Autodesk Fusion 360 part; units mm, degrees
note: some values were not read from the file. Chosen so that the rebuilt part matches the saved one: which bodies a step acts on.
(part 2 of 2)
  arc A177 (168.3933, -28.1734) -> (169.3933, -29.1734) centre (169.3933, -28.1734) ccw
  arc A178 (168.3933, -28.1734) -> (169.3933, -29.1734) centre (169.3933, -28.1734) ccw
  line L233 (31.4836, -7.7355) -> (36.2443, -10.861)
  line L234 (10.9623, -64.1171) -> (5.4942, -62.1268)
  line L235 (96.3933, -30.1734) -> (89.3933, -30.1734)
  line L236 (5.4942, -62.1268) -> (22.5952, -15.1422)
  line L237 (410.3933, -50.1734) -> (410.3933, -48.1734)
  arc A179 (386.6208, -12.1734) -> (390.6208, -16.1734) centre (386.6208, -16.1734) cw
  arc A180 (88.3933, -33.1734) -> (89.3933, -34.1734) centre (89.3933, -33.1734) ccw
  arc A181 (386.6208, -12.1734) -> (390.6208, -16.1734) centre (386.6208, -16.1734) cw
  line L238 (401.3933, -58.1734) -> (401.3933, -60.1734)
  arc A182 (96.3933, -34.1734) -> (97.3933, -33.1734) centre (96.3933, -33.1734) ccw
  arc A183 (88.3933, -23.1734) -> (89.3933, -24.1734) centre (89.3933, -23.1734) ccw
  line L239 (28.0509, -66.2863) -> (7.5421, -73.514)
  arc A184 (402.3933, -47.1734) -> (401.3933, -48.1734) centre (402.3933, -48.1734) ccw
  arc A185 (176.3933, -29.1734) -> (177.3933, -28.1734) centre (176.3933, -28.1734) ccw
  line L240 (177.3933, -22.1734) -> (177.3933, -16.1734)
  line L241 (168.3933, -22.1734) -> (168.3933, -16.1734)
  arc A186 (108.1658, -53.1734) -> (112.1658, -49.1734) centre (112.1658, -53.1734) cw
  line L242 (169.3933, -29.1734) -> (176.3933, -29.1734)
  line L243 (410.3933, -50.1734) -> (410.3933, -48.1734)
  line L244 (89.3933, -34.1734) -> (96.3933, -34.1734)
  line L245 (28.0633, -17.1324) -> (31.4836, -7.7355)
  line L246 (696.9999, -83.525) -> (3, -83.525)
  line L247 (683.9505, -160) -> (683.9505, -210)
  line L248 (680.9505, -160) -> (683.9505, -160)
  line L249 (40.6348, -12.1734) -> (386.6208, -12.1734)
  arc A187 (227.4798, -32.1734) -> (28.0509, -66.2863) centre (227.4798, -632.1734) ccw
  line L250 (458.1519, -69.1734) -> (112.1658, -69.1734)
  line L251 (321.3933, -59.1734) -> (321.3933, -65.1734)
  line L252 (402.3933, -51.1734) -> (409.3933, -51.1734)
  line L253 (21.9994, -210) -> (21.9994, -160)
  arc A188 (402.3933, -57.1734) -> (401.3933, -58.1734) centre (402.3933, -58.1734) ccw
  line L254 (22.5952, -15.1422) -> (28.0633, -17.1324)
  line L255 (168.3933, -22.1734) -> (168.3933, -28.1734)
  arc A189 (409.3933, -61.1734) -> (410.3933, -60.1734) centre (409.3933, -60.1734) ccw
  line L256 (88.3933, -23.1734) -> (88.3933, -21.1734)
  arc A190 (329.3933, -66.1734) -> (330.3933, -65.1734) centre (329.3933, -65.1734) ccw
  line L257 (169.3933, -15.1734) -> (176.3933, -15.1734)
  line L258 (21.9994, -160) -> (19.0494, -160)
  line L259 (19.0494, -210) -> (21.9994, -210)
  arc A191 (329.3933, -66.1734) -> (330.3933, -65.1734) centre (329.3933, -65.1734) ccw
  line L260 (88.3933, -31.1734) -> (88.3933, -33.1734)
  line L261 (487.8243, -17.2297) -> (493.2925, -19.2199)
  arc A192 (3, -83.525) -> (0, -86.525) centre (3, -86.525) ccw
  line L262 (329.3933, -52.1734) -> (322.3933, -52.1734)
  arc A193 (410.3933, -48.1734) -> (409.3933, -47.1734) centre (409.3933, -48.1734) ccw
  line L263 (329.3933, -66.1734) -> (322.3933, -66.1734)
  line L264 (402.3933, -57.1734) -> (409.3933, -57.1734)
  arc A194 (410.3933, -58.1734) -> (409.3933, -57.1734) centre (409.3933, -58.1734) ccw
  line L265 (7.5421, -73.514) -> (10.9623, -64.1171)
  line L266 (321.3933, -59.1734) -> (321.3933, -53.1734)
  line L267 (491.2445, -7.8327) -> (487.8243, -17.2297)
  arc A195 (321.3933, -65.1734) -> (322.3933, -66.1734) centre (322.3933, -65.1734) ccw
  line L268 (493.2925, -19.2199) -> (476.1915, -66.2045)
  arc A196 (177.3933, -16.1734) -> (176.3933, -15.1734) centre (176.3933, -16.1734) ccw
  arc A197 (402.3933, -47.1734) -> (401.3933, -48.1734) centre (402.3933, -48.1734) ccw
  line L269 (329.3933, -52.1734) -> (322.3933, -52.1734)
  line L270 (177.3933, -22.1734) -> (177.3933, -28.1734)
  line L271 (470.7233, -64.2143) -> (467.3031, -73.6112)
  line L272 (96.3933, -24.1734) -> (89.3933, -24.1734)
  line L273 (329.3933, -66.1734) -> (322.3933, -66.1734)
  line L274 (168.3933, -22.1734) -> (168.3933, -28.1734)
  arc A198 (462.5423, -70.4858) -> (458.1519, -69.1734) centre (458.1519, -77.1734) ccw
  arc A199 (88.3933, -33.1734) -> (89.3933, -34.1734) centre (89.3933, -33.1734) ccw
  line L275 (330.3933, -59.1734) -> (330.3933, -65.1734)
  arc A200 (96.3933, -24.1734) -> (97.3933, -23.1734) centre (96.3933, -23.1734) ccw
  arc A201 (322.3933, -52.1734) -> (321.3933, -53.1734) centre (322.3933, -53.1734) ccw
  arc A202 (88.3933, -23.1734) -> (89.3933, -24.1734) centre (89.3933, -23.1734) ccw
  arc A203 (169.3933, -15.1734) -> (168.3933, -16.1734) centre (169.3933, -16.1734) ccw
  arc A204 (176.3933, -29.1734) -> (177.3933, -28.1734) centre (176.3933, -28.1734) ccw
  arc A205 (321.3933, -65.1734) -> (322.3933, -66.1734) centre (322.3933, -65.1734) ccw
  line L276 (89.3933, -20.1734) -> (96.3933, -20.1734)
  line L277 (330.3933, -59.1734) -> (330.3933, -53.1734)
  arc A206 (390.6208, -28.1734) -> (386.6208, -32.1734) centre (386.6208, -28.1734) cw
  arc A207 (36.2443, -10.861) -> (40.6348, -12.1734) centre (40.6348, -4.1734) ccw
  arc A208 (401.3933, -60.1734) -> (402.3933, -61.1734) centre (402.3933, -60.1734) ccw
  arc A209 (89.3933, -20.1734) -> (88.3933, -21.1734) centre (89.3933, -21.1734) ccw
  line L278 (321.3933, -59.1734) -> (321.3933, -53.1734)
  arc A210 (177.3933, -16.1734) -> (176.3933, -15.1734) centre (176.3933, -16.1734) ccw
  line L279 (112.1658, -49.1734) -> (271.3069, -49.1734)
  line L280 (680.9505, -210) -> (678.0005, -210)
  arc A211 (696.9999, -220) -> (699.9999, -217) centre (696.9999, -217) ccw
  line L281 (678.0005, -160) -> (680.9505, -160)
  line L282 (458.1519, -69.1734) -> (112.1658, -69.1734)
  line L283 (3, -220) -> (696.9999, -220)
  line L284 (386.6208, -32.1734) -> (227.4798, -32.1734)
  arc A212 (227.4798, -32.1734) -> (28.0509, -66.2863) centre (227.4798, -632.1734) ccw
  line L285 (386.6208, -32.1734) -> (227.4798, -32.1734)
  arc A213 (271.3069, -49.1734) -> (470.7357, -15.0604) centre (271.3069, 550.8266) ccw
  arc A214 (271.3069, -49.1734) -> (470.7357, -15.0604) centre (271.3069, 550.8266) ccw
  line L286 (0, -86.525) -> (0, -217)
  line L287 (96.3933, -24.1734) -> (89.3933, -24.1734)
  arc A215 (699.9999, -86.525) -> (696.9999, -83.525) centre (696.9999, -86.525) ccw
  line L288 (699.9999, -217) -> (699.9999, -86.525)
  line L289 (470.7357, -15.0604) -> (491.2445, -7.8327)
  line L290 (491.2445, -7.8327) -> (487.8243, -17.2297)
  arc A216 (97.3933, -21.1734) -> (96.3933, -20.1734) centre (96.3933, -21.1734) ccw
  line L291 (402.3933, -57.1734) -> (409.3933, -57.1734)
  line L292 (97.3933, -23.1734) -> (97.3933, -21.1734)
  arc A217 (322.3933, -52.1734) -> (321.3933, -53.1734) centre (322.3933, -53.1734) ccw
  arc A218 (89.3933, -30.1734) -> (88.3933, -31.1734) centre (89.3933, -31.1734) ccw
  arc A219 (112.1658, -69.1734) -> (108.1658, -65.1734) centre (112.1658, -65.1734) cw
  line L293 (493.2925, -19.2199) -> (476.1915, -66.2045)
  line L294 (16.0494, -210) -> (19.0494, -210)
  line L295 (467.3031, -73.6112) -> (462.5423, -70.4858)
  arc A220 (330.3933, -53.1734) -> (329.3933, -52.1734) centre (329.3933, -53.1734) ccw
  line L296 (108.1658, -65.1734) -> (108.1658, -53.1734)
  line L297 (467.3031, -73.6112) -> (462.5423, -70.4858)
  line L298 (97.3933, -23.1734) -> (97.3933, -21.1734)
  arc A221 (0, -217) -> (3, -220) centre (3, -217) ccw
  line L299 (470.7357, -15.0604) -> (491.2445, -7.8327)
  line L300 (409.3933, -47.1734) -> (402.3933, -47.1734)
  line L301 (487.8243, -17.2297) -> (493.2925, -19.2199)
  line L302 (108.1658, -65.1734) -> (108.1658, -53.1734)
  line L303 (476.1915, -66.2045) -> (470.7233, -64.2143)
  line L304 (97.3933, -31.1734) -> (97.3933, -33.1734)
  arc A222 (401.3933, -50.1734) -> (402.3933, -51.1734) centre (402.3933, -50.1734) ccw
  line L305 (330.3933, -59.1734) -> (330.3933, -65.1734)
  arc A223 (97.3933, -31.1734) -> (96.3933, -30.1734) centre (96.3933, -31.1734) ccw
  line L306 (19.0494, -160) -> (16.0494, -160)
  arc A224 (108.1658, -53.1734) -> (112.1658, -49.1734) centre (112.1658, -53.1734) cw
  line L307 (321.3933, -59.1734) -> (321.3933, -65.1734)
  line L308 (409.3933, -47.1734) -> (402.3933, -47.1734)
  arc A225 (462.5423, -70.4858) -> (458.1519, -69.1734) centre (458.1519, -77.1734) ccw
  line L309 (470.7233, -64.2143) -> (467.3031, -73.6112)
  arc A226 (330.3933, -53.1734) -> (329.3933, -52.1734) centre (329.3933, -53.1734) ccw
  line L310 (330.3933, -59.1734) -> (330.3933, -53.1734)
  line L311 (476.1915, -66.2045) -> (470.7233, -64.2143)
  line L312 (89.3933, -34.1734) -> (96.3933, -34.1734)
  arc A227 (390.6208, -28.1734) -> (386.6208, -32.1734) centre (386.6208, -28.1734) cw
  arc A228 (112.1658, -69.1734) -> (108.1658, -65.1734) centre (112.1658, -65.1734) cw
  arc A229 (401.3933, -50.1734) -> (402.3933, -51.1734) centre (402.3933, -50.1734) ccw
  arc A230 (401.3933, -60.1734) -> (402.3933, -61.1734) centre (402.3933, -60.1734) ccw
  line L313 (16.0494, -160) -> (16.0494, -210)
  line L314 (683.9505, -210) -> (680.9505, -210)
  line L315 (678.0005, -210) -> (678.0005, -160)
  line L316 (39.1156, -28.6044) -> (42.6539, -25.6355)
  line L317 (42.6539, -25.6355) -> (41.8518, -21.0869)
  line L318 (41.8518, -21.0869) -> (37.5116, -19.5071)
  line L319 (37.5116, -19.5071) -> (33.9733, -22.476)
  line L320 (33.9733, -22.476) -> (34.7754, -27.0247)
  line L321 (34.7754, -27.0247) -> (39.1156, -28.6044)
  line L322 (28.171, -58.6746) -> (31.7092, -55.7056)
  line L323 (31.7092, -55.7056) -> (30.9072, -51.157)
  line L324 (30.9072, -51.157) -> (26.5669, -49.5773)
  line L325 (26.5669, -49.5773) -> (23.0287, -52.5462)
  line L326 (23.0287, -52.5462) -> (23.8307, -57.0948)
  line L327 (23.8307, -57.0948) -> (28.171, -58.6746)
  line L328 (461.2751, -61.8396) -> (464.8133, -58.8707)
  line L329 (464.8133, -58.8707) -> (464.0113, -54.3221)
  line L330 (464.0113, -54.3221) -> (459.671, -52.7423)
  line L331 (459.671, -52.7423) -> (456.1328, -55.7113)
  line L332 (456.1328, -55.7113) -> (456.9349, -60.2599)
  line L333 (456.9349, -60.2599) -> (461.2751, -61.8396)
  line L334 (472.2197, -31.7695) -> (475.758, -28.8005)
  line L335 (475.758, -28.8005) -> (474.9559, -24.2519)
  line L336 (474.9559, -24.2519) -> (470.6157, -22.6722)
  line L337 (470.6157, -22.6722) -> (467.0774, -25.6411)
  line L338 (467.0774, -25.6411) -> (467.8795, -30.1897)
  line L339 (467.8795, -30.1897) -> (472.2197, -31.7695)
  line L340 (206.5688, -24.9234) -> (208.1565, -22.1734)
  line L341 (208.1565, -22.1734) -> (206.5688, -19.4234)
  line L342 (206.5688, -19.4234) -> (203.3934, -19.4234)
  line L343 (203.3934, -19.4234) -> (201.8057, -22.1734)
  line L344 (201.8057, -22.1734) -> (203.3934, -24.9234)
  line L345 (203.3934, -24.9234) -> (206.5688, -24.9234)
  line L346 (278.5688, -24.9234) -> (280.1565, -22.1734)
  line L347 (280.1565, -22.1734) -> (278.5688, -19.4234)
  line L348 (278.5688, -19.4234) -> (275.3934, -19.4234)
  line L349 (275.3934, -19.4234) -> (273.8057, -22.1734)
  line L350 (273.8057, -22.1734) -> (275.3934, -24.9234)
  line L351 (275.3934, -24.9234) -> (278.5688, -24.9234)
  line L352 (350.5688, -24.9234) -> (352.1565, -22.1734)
  line L353 (352.1565, -22.1734) -> (350.5688, -19.4234)
  line L354 (350.5688, -19.4234) -> (347.3934, -19.4234)
  line L355 (347.3934, -19.4234) -> (345.8057, -22.1734)
  line L356 (345.8057, -22.1734) -> (347.3934, -24.9234)
  line L357 (347.3934, -24.9234) -> (350.5688, -24.9234)
  line L358 (295.3933, -61.9234) -> (296.981, -59.1734)
  line L359 (296.981, -59.1734) -> (295.3933, -56.4234)
  line L360 (295.3933, -56.4234) -> (292.2178, -56.4234)
  line L361 (292.2178, -56.4234) -> (290.6301, -59.1734)
  line L362 (290.6301, -59.1734) -> (292.2178, -61.9234)
  line L363 (292.2178, -61.9234) -> (295.3933, -61.9234)
  line L364 (223.3933, -61.9234) -> (224.981, -59.1734)
  line L365 (224.981, -59.1734) -> (223.3933, -56.4234)
  line L366 (223.3933, -56.4234) -> (220.2178, -56.4234)
  line L367 (220.2178, -56.4234) -> (218.6301, -59.1734)
  line L368 (218.6301, -59.1734) -> (220.2178, -61.9234)
  line L369 (220.2178, -61.9234) -> (223.3933, -61.9234)
  line L370 (151.3933, -61.9234) -> (152.981, -59.1734)
  line L371 (152.981, -59.1734) -> (151.3933, -56.4234)
  line L372 (151.3933, -56.4234) -> (148.2178, -56.4234)
  line L373 (148.2178, -56.4234) -> (146.6301, -59.1734)
  line L374 (146.6301, -59.1734) -> (148.2178, -61.9234)
  line L375 (148.2178, -61.9234) -> (151.3933, -61.9234)
  line L376 (351.5896, -105.525) -> (353.1773, -102.775)
  line L377 (353.1773, -102.775) -> (351.5896, -100.025)
  line L378 (351.5896, -100.025) -> (348.4142, -100.025)
  line L379 (348.4142, -100.025) -> (346.8265, -102.775)
  line L380 (346.8265, -102.775) -> (348.4142, -105.525)
  line L381 (348.4142, -105.525) -> (351.5896, -105.525)
  line L382 (348.4142, -213.025) -> (346.8265, -215.775)
  line L383 (346.8265, -215.775) -> (348.4142, -218.525)
  line L384 (348.4142, -218.525) -> (351.5896, -218.525)
  line L385 (351.5896, -218.525) -> (353.1773, -215.775)
  line L386 (353.1773, -215.775) -> (351.5896, -213.025)
  line L387 (351.5896, -213.025) -> (348.4142, -213.025)
  line L388 (593.6142, -213.025) -> (592.0265, -215.775)
  line L389 (592.0265, -215.775) -> (593.6142, -218.525)
  line L390 (593.6142, -218.525) -> (596.7896, -218.525)
  line L391 (596.7896, -218.525) -> (598.3773, -215.775)
  line L392 (598.3773, -215.775) -> (596.7896, -213.025)
  line L393 (596.7896, -213.025) -> (593.6142, -213.025)
  line L394 (595.1127, -162.375) -> (596.7004, -159.625)
  line L395 (596.7004, -159.625) -> (595.1127, -156.875)
  line L396 (595.1127, -156.875) -> (591.9373, -156.875)
  line L397 (591.9373, -156.875) -> (590.3496, -159.625)
  line L398 (590.3496, -159.625) -> (591.9373, -162.375)
  line L399 (591.9373, -162.375) -> (595.1127, -162.375)
  line L400 (570.7896, -99.525) -> (572.3773, -96.775)
  line L401 (572.3773, -96.775) -> (570.7896, -94.025)
  line L402 (570.7896, -94.025) -> (567.6142, -94.025)
  line L403 (567.6142, -94.025) -> (566.0265, -96.775)
  line L404 (566.0265, -96.775) -> (567.6142, -99.525)
  line L405 (567.6142, -99.525) -> (570.7896, -99.525)
  line L406 (132.5896, -99.525) -> (134.1773, -96.775)
  line L407 (134.1773, -96.775) -> (132.5896, -94.025)
  line L408 (132.5896, -94.025) -> (129.4142, -94.025)
  line L409 (129.4142, -94.025) -> (127.8265, -96.775)
  line L410 (127.8265, -96.775) -> (129.4142, -99.525)
  line L411 (129.4142, -99.525) -> (132.5896, -99.525)
  line L412 (108.0627, -162.375) -> (109.6504, -159.625)
  line L413 (109.6504, -159.625) -> (108.0627, -156.875)
  line L414 (108.0627, -156.875) -> (104.8873, -156.875)
  line L415 (104.8873, -156.875) -> (103.2996, -159.625)
  line L416 (103.2996, -159.625) -> (104.8873, -162.375)
  line L417 (104.8873, -162.375) -> (108.0627, -162.375)
  line L418 (103.4142, -213.025) -> (101.8265, -215.775)
  line L419 (101.8265, -215.775) -> (103.4142, -218.525)
  line L420 (103.4142, -218.525) -> (106.5896, -218.525)
  line L421 (106.5896, -218.525) -> (108.1773, -215.775)
  line L422 (108.1773, -215.775) -> (106.5896, -213.025)
  line L423 (106.5896, -213.025) -> (103.4142, -213.025)
  line L424 (36.2593, -211) -> (38.5687, -207)
  line L425 (38.5687, -207) -> (36.2593, -203)
  line L426 (36.2593, -203) -> (31.6405, -203)
  line L427 (31.6405, -203) -> (29.3311, -207)
  line L428 (29.3311, -207) -> (31.6405, -211)
  line L429 (31.6405, -211) -> (36.2593, -211)
  line L430 (36.2593, -179) -> (38.5687, -175)
  line L431 (38.5687, -175) -> (36.2593, -171)
  line L432 (36.2593, -171) -> (31.6405, -171)
  line L433 (31.6405, -171) -> (29.3311, -175)
  line L434 (29.3311, -175) -> (31.6405, -179)
  line L435 (31.6405, -179) -> (36.2593, -179)
  line L436 (668.3594, -211) -> (670.6688, -207)
  line L437 (670.6688, -207) -> (668.3594, -203)
  line L438 (668.3594, -203) -> (663.7406, -203)
  line L439 (663.7406, -203) -> (661.4312, -207)
  line L440 (661.4312, -207) -> (663.7406, -211)
  line L441 (663.7406, -211) -> (668.3594, -211)
  line L442 (668.3594, -179) -> (670.6688, -175)
  line L443 (670.6688, -175) -> (668.3594, -171)
  line L444 (668.3594, -171) -> (663.7406, -171)
  line L445 (663.7406, -171) -> (661.4312, -175)
  line L446 (661.4312, -175) -> (663.7406, -179)
  line L447 (663.7406, -179) -> (668.3594, -179)
  line L448 (349.9999, 68.2375) -> (351, 68.2375)
  line L449 (370, 87.2375) -> (370, 136.475)
  line L450 (349.9999, 68.2375) -> (349, 68.2375)
  line L451 (330, 49.2375) -> (330, 0)
  line L452 (349.9999, -151.7625) -> (351, -151.7625)
  line L453 (370, -132.7625) -> (370, -83.525)
  line L454 (349.9999, -151.7625) -> (349, -151.7625)
  line L455 (330, -170.7625) -> (330, -220)
  arc A231 (349, -151.7625) -> (330, -170.7625) centre (349, -170.7625) ccw
  arc A232 (351, -151.7625) -> (370, -132.7625) centre (351, -132.7625) ccw
  arc A233 (349, 68.2375) -> (330, 49.2375) centre (349, 49.2375) ccw
  arc A234 (351, 68.2375) -> (370, 87.2375) centre (351, 87.2375) ccw
  point P0 (0, 136.475)
  point P1 (0, 136.475)
  point P2 (0, -220)
  point P3 (0, -220)
  point P4 (0, -220)
  point P5 (0, -83.525)
  point P6 (38.3136, -24.0558)
  point P7 (27.369, -54.1259)
  point P8 (460.4731, -57.291)
  point P9 (471.4177, -27.2208)
  point P10 (204.9811, -22.1734)
  point P11 (276.9811, -22.1734)
  point P12 (348.9811, -22.1734)
  point P13 (293.8055, -59.1734)
  point P14 (221.8055, -59.1734)
  point P15 (149.8055, -59.1734)
  point P16 (350.0019, -102.775)
  point P17 (350.0019, -215.775)
  point P18 (595.2019, -215.775)
  point P19 (593.525, -159.625)
  point P20 (569.2019, -96.775)
  point P21 (131.0019, -96.775)
  point P22 (106.475, -159.625)
  point P23 (105.0019, -215.775)
  point P24 (33.9499, -207)
  point P25 (33.9499, -175)
  point P26 (666.05, -207)
  point P27 (666.05, -175)
  dimension "d111" = 136.475
  dimension "d112" = 3
  dimension "d113" = 3
  dimension "d114" = 3
  dimension "d115" = 3
  dimension "d116" = 3
  dimension "d117" = 3
  dimension "d118" = 3
  dimension "d119" = 3
  dimension "d120" = 3
  dimension "d121" = 1
  dimension "d122" = 1
  dimension "d123" = 1
  dimension "d124" = 1
  dimension "d125" = 136.475
  dimension "d126" = 3
  dimension "d127" = 3
  dimension "d128" = 3
  dimension "d129" = 3
  dimension "d130" = 3
  dimension "d131" = 3
  dimension "d132" = 3
  dimension "d133" = 3
  dimension "d134" = 3
  dimension "d135" = 1
  dimension "d136" = 1
  dimension "d137" = 1
  dimension "d138" = 1
  dimension "d139" = 136.475
  dimension "d140" = 3
  dimension "d149" = 1
  dimension "d150" = 1
  dimension "d151" = 1
  dimension "d152" = 1
  dimension "d153" = 4
  dimension "d154" = 4
  dimension "d155" = 4
  dimension "d156" = 4
  dimension "d157" = 2.75
  dimension "d158" = 2.75
  dimension "d159" = 2.75
  dimension "d160" = 2.75
  dimension "d161" = 2.75
  dimension "d162" = 2.75
  dimension "d163" = 2.75
  dimension "d164" = 2.75
  dimension "d165" = 2.75
  dimension "d166" = 2.75
  dimension "d167" = 2.75
  dimension "d168" = 4
  dimension "d169" = 4
  dimension "d170" = 4
  dimension "d171" = 4
  dimension "d172" = 19
  dimension "d173" = 19
  constraint horizontal L0
  constraint vertical L2
  constraint horizontal L1
  constraint vertical L3
  constraint tangent L2 A9
  constraint tangent L1 A9
  constraint tangent L0 A5
  constraint tangent L2 A5
  constraint equal A5 A9
  constraint coincident origin L0
  constraint coincident origin L3
  constraint tangent L0 A4
  constraint tangent A4 L3
  constraint equal A4 A9
  constraint coincident P1 L1
  constraint coincident P1 L3
  constraint tangent L1 A11
  constraint tangent L3 A11
  constraint equal A9 A11
  constraint perpendicular L21 L26
  constraint perpendicular L22 L27
  constraint tangent L27 A26
  constraint tangent L22 A26
  constraint tangent L27 A27
  constraint tangent L24 A27
  constraint equal A26 A27
  constraint tangent L26 A28
  constraint tangent L25 A28
  constraint equal A26 A28
  constraint tangent L26 A29
  constraint tangent L21 A29
  constraint equal A26 A29
  constraint perpendicular L36 L44
  constraint perpendicular L32 L37
  constraint tangent L37 A45
  constraint tangent L32 A45
  constraint tangent L37 A34
  constraint tangent A34 L41
  constraint equal A34 A45
  constraint tangent L36 A42
  constraint tangent L39 A42
  constraint equal A42 A45
  constraint tangent A31 L36
  constraint tangent A31 L44
  constraint equal A31 A45
  constraint perpendicular L69 L71
  constraint perpendicular L72 L76
  constraint tangent L72 A72
  constraint tangent A72 L76
  constraint tangent L72 A66
  constraint tangent L62 A66
  constraint equal A66 A72
  constraint tangent L69 A68
  constraint tangent A68 L96
  constraint equal A68 A72
  constraint tangent L69 A71
  constraint tangent L71 A71
  constraint equal A71 A72
  constraint perpendicular L63 L68
  constraint perpendicular L51 L64
  constraint tangent L64 A59
  constraint tangent L51 A59
  constraint tangent A52 L64
  constraint tangent A52 L86
  constraint equal A52 A59
  constraint tangent L63 A60
  constraint tangent L53 A60
  constraint equal A59 A60
  constraint tangent A50 L63
  constraint tangent A50 L68
  constraint equal A50 A59
  constraint horizontal L177
  constraint vertical L180
  constraint horizontal L145
  constraint vertical L178
  constraint tangent A139 L180
  constraint tangent L145 A139
  constraint tangent A133 L177
  constraint tangent A133 L180
  constraint equal A133 A139
  constraint coincident origin L177
  constraint coincident origin L178
  constraint tangent L177 A149
  constraint tangent L178 A149
  constraint equal A139 A149
  constraint coincident P1 L145
  constraint coincident P1 L178
  constraint tangent L145 A112
  constraint tangent A112 L178
  constraint equal A112 A139
  constraint perpendicular L112 L117
  constraint perpendicular L137 L183
  constraint tangent A89 L183
  constraint tangent A89 L137
  constraint tangent A86 L183
  constraint tangent L107 A86
  constraint equal A86 A89
  constraint tangent A88 L117
  constraint tangent A88 L142
  constraint equal A88 A89
  constraint tangent L117 A159
  constraint tangent L112 A159
  constraint equal A89 A159
  constraint perpendicular L129 L150
  constraint perpendicular L118 L160
  constraint tangent A107 L160
  constraint tangent L118 A107
  constraint tangent L160 A114
  constraint tangent L114 A114
  constraint equal A107 A114
  constraint tangent A83 L150
  constraint tangent A83 L136
  constraint equal A83 A107
  constraint tangent L150 A151
  constraint tangent L129 A151
  constraint equal A107 A151
  constraint perpendicular L134 L196
  constraint perpendicular L168 L184
  constraint tangent L168 A121
  constraint tangent A121 L184
  constraint tangent L168 A123
  constraint tangent L106 A123
  constraint equal A121 A123
  constraint tangent L134 A145
  constraint tangent L121 A145
  constraint equal A121 A145
  constraint tangent L134 A152
  constraint tangent L196 A152
  constraint equal A121 A152
  constraint perpendicular L122 L124
  constraint perpendicular L179 L190
  constraint tangent A82 L179
  constraint tangent A82 L190
  constraint tangent A100 L179
  constraint tangent A100 L154
  constraint equal A82 A100
  constraint tangent L124 A92
  constraint tangent A92 L156
  constraint equal A82 A92
  constraint tangent A91 L124
  constraint tangent L122 A91
  constraint equal A82 A91
  constraint horizontal L283
  constraint vertical L288
  constraint horizontal L246
  constraint vertical L286
  constraint coincident P4 P3
  constraint tangent A215 L288
  constraint tangent L246 A215
  constraint tangent A211 L283
  constraint tangent A211 L288
  constraint equal A211 A215
  constraint coincident P4 L283
  constraint coincident P4 L286
  constraint tangent L283 A221
  constraint tangent L286 A221
  constraint equal A215 A221
  constraint coincident P5 L246
  constraint coincident P5 L286
  constraint tangent L246 A192
  constraint tangent A192 L286
  constraint equal A192 A215
  constraint perpendicular L213 L218
  constraint perpendicular L238 L291
  constraint tangent A170 L291
  constraint tangent A170 L238
  constraint tangent A167 L291
  constraint tangent L207 A167
  constraint equal A167 A170
  constraint tangent A169 L218
  constraint tangent A169 L243
  constraint equal A169 A170
  constraint tangent L218 A229
  constraint tangent L213 A229
  constraint equal A170 A229
  constraint perpendicular L230 L252
  constraint perpendicular L219 L264
  constraint tangent A188 L264
  constraint tangent L219 A188
  constraint tangent L264 A194
  constraint tangent L215 A194
  constraint equal A188 A194
  constraint tangent A164 L252
  constraint tangent A164 L237
  constraint equal A164 A188
  constraint tangent L252 A222
  constraint tangent L230 A222
  constraint equal A188 A222
  constraint perpendicular L235 L304
  constraint perpendicular L272 L292
  constraint tangent L272 A200
  constraint tangent A200 L292
  constraint tangent L272 A202
  constraint tangent L206 A202
  constraint equal A200 A202
  constraint tangent L235 A218
  constraint tangent L222 A218
  constraint equal A200 A218
  constraint tangent L235 A223
  constraint tangent L304 A223
  constraint equal A200 A223
  constraint perpendicular L223 L225
  constraint perpendicular L287 L298
  constraint tangent A163 L287
  constraint tangent A163 L298
  constraint tangent A183 L287
  constraint tangent A183 L256
  constraint equal A163 A183
  constraint tangent L225 A173
  constraint tangent A173 L260
  constraint equal A163 A173
  constraint tangent A172 L225
  constraint tangent L223 A172
  constraint equal A163 A172
  constraint coincident L1 L449.end
  constraint perpendicular L1 L449
  constraint coincident L0 L451.end
  constraint perpendicular L0 L451
  constraint coincident L246 L453.end
  constraint perpendicular L246 L453
  constraint coincident L283 L455.end
  constraint perpendicular L283 L455
  constraint tangent L454 A231
  constraint tangent L455 A231
  constraint tangent L452 A232
  constraint tangent L453 A232
  constraint equal A231 A232
  constraint tangent L450 A233
  constraint tangent L451 A233
  constraint tangent L448 A234
  constraint tangent L449 A234
  constraint equal A233 A234
  measures "d111" distance of origin P1
  measures "d112" radius of A9
  measures "d113" diameter of A7
  measures "d114" diameter of A6
  measures "d115" diameter of A3
  measures "d116" diameter of A10
  measures "d117" diameter of A2
  measures "d118" diameter of A1
  measures "d119" diameter of A8
  measures "d120" diameter of A0
  measures "d121" radius of A26
  measures "d122" radius of A45
  measures "d123" radius of A72
  measures "d124" radius of A59
  measures "d125" distance of origin P1
  measures "d126" radius of A139
  measures "d127" diameter of A140
  measures "d128" diameter of A138
  measures "d129" diameter of A137
  measures "d130" diameter of A135
  measures "d131" diameter of A106
  measures "d132" diameter of A162
  measures "d133" diameter of A150
  measures "d134" diameter of A131
  measures "d135" radius of A89
  measures "d136" radius of A107
  measures "d137" radius of A121
  measures "d138" radius of A82
  measures "d139" distance of P4 P5
  measures "d140" radius of A215
  measures "d149" radius of A170
  measures "d150" radius of A188
  measures "d151" radius of A200
  measures "d152" radius of A163
  measures "d153" distance of P6 L321
  measures "d154" distance of P7 L327
  measures "d155" distance of P8 L333
  measures "d156" distance of P9 L339
  measures "d157" distance of P10 L345
  measures "d158" distance of P11 L351
  measures "d159" distance of P13 L363
  measures "d160" distance of P16 L381
  measures "d161" distance of P17 L387
  measures "d162" distance of P18 L393
  measures "d163" distance of P19 L399
  measures "d164" distance of P20 L405
  measures "d165" distance of P21 L411
  measures "d166" distance of P22 L417
  measures "d167" distance of P23 L423
  measures "d168" distance of P24 L429
  measures "d169" distance of P25 L435
  measures "d170" distance of P26 L441
  measures "d171" distance of P27 L447
  measures "d172" radius of A231
  measures "d173" radius of A233
sketch "PCB Backplate" plane through (0, 0, 0) normal (0, 1, 0) x (1, 0, 0)
  circle A0 centre (469.2019, 123.225) radius 1.5
  arc A1 (454, 109) -> (457, 112) centre (454, 112) ccw
  arc A2 (486.0019, 133.475) -> (483.0019, 136.475) centre (483.0019, 133.475) ccw
  line L0 (496.9999, 111) -> (489.0019, 111)
  arc A3 (457, 118) -> (454, 121) centre (454, 118) ccw
  line L1 (3, 0) -> (497.0008, 0)
  line L2 (394, 136.475) -> (17, 136.475)
  line L3 (486.0019, 114) -> (486.0019, 133.475)
  arc A4 (434.5275, 124) -> (437.5275, 121) centre (437.5275, 124) ccw
  arc A5 (11, 111) -> (14, 114) centre (11, 114) ccw
  line L4 (451.25, 19.35) -> (441.1364, 19.35) construction
  arc A6 (397, 112) -> (400, 109) centre (400, 112) ccw
  circle A7 centre (31, 123.225) radius 1.5
  line L5 (434.5275, 133.475) -> (434.5275, 124)
  line L6 (0, 108) -> (0, 3)
  line L7 (499.9999, 2.9991) -> (499.9999, 108)
  arc A8 (3, 111) -> (0, 108) centre (3, 108) ccw
  line L8 (437.5275, 121) -> (454, 121)
  line L9 (483.0019, 136.475) -> (437.5275, 136.475)
  line L10 (3, 111) -> (11, 111)
  line L11 (454, 109) -> (400, 109)
  circle A9 centre (5.0019, 4.225) radius 1.5
  circle A10 centre (495.2019, 4.225) radius 1.5
  arc A11 (497.0008, 0) -> (499.9999, 2.9991) centre (497.0008, 2.9991) ccw
  circle A12 centre (250.0019, 117.225) radius 1.5
  circle A13 centre (6.475, 60.35) radius 1.5
  circle A14 centre (6.475, 60.375) radius 1.5
  arc A15 (0, 3) -> (3, 0) centre (3, 3) ccw
  circle A16 centre (250.0019, 4.225) radius 1.5
  circle A17 centre (493.525, 60.375) radius 1.5
  arc A18 (17, 136.475) -> (14, 133.475) centre (17, 133.475) ccw
  line L12 (14, 114) -> (14, 133.475)
  arc A19 (397, 133.475) -> (394, 136.475) centre (394, 133.475) ccw
  line L13 (397, 112) -> (397, 133.475)
  circle A20 centre (31.0019, 123.225) radius 1.5
  arc A21 (437.5275, 136.475) -> (434.5275, 133.475) centre (437.5275, 133.475) ccw
  line L14 (457, 118) -> (457, 112)
  arc A22 (486.0019, 114) -> (489.0019, 111) centre (489.0019, 114) ccw
  arc A23 (499.9999, 108) -> (496.9999, 111) centre (496.9999, 108) ccw
  line L15 (451.25, 19.35) -> (439.25, 19.35) construction
  line L16 (472, 17) -> (24.4885, 17)
  line L17 (24.4885, 17) -> (24.4885, 10.5)
  line L18 (24.4885, 10.5) -> (472, 10.5)
  line L19 (472, 10.5) -> (472, 17)
  line L20 (94, 130.5) -> (110.5, 130.5)
  line L21 (110.5, 130.5) -> (110.5, 122.5)
  line L22 (110.5, 122.5) -> (94, 122.5)
  line L23 (94, 122.5) -> (94, 130.5)
  line L24 (336.8, 130.5) -> (353.3, 130.5)
  line L25 (353.3, 130.5) -> (353.3, 122.5)
  line L26 (353.3, 122.5) -> (336.8, 122.5)
  line L27 (336.8, 122.5) -> (336.8, 130.5)
  point P0 (0, 136.475)
  dimension "d178" = 136.475
  dimension "d179" = 3
  dimension "d180" = 3
  dimension "d181" = 3
  dimension "d182" = 3
  dimension "d183" = 3
  dimension "d184" = 3
  dimension "d185" = 3
  dimension "d186" = 3
  dimension "d190" = 3
  dimension "d191" = 3
  constraint horizontal L1
  constraint vertical L7
  constraint horizontal L9
  constraint vertical L6
  constraint tangent L1 A11
  constraint tangent L7 A11
  constraint coincident origin L1
  constraint coincident origin L6
  constraint tangent L1 A15
  constraint tangent L6 A15
  constraint coincident P0 L2
  constraint coincident P0 L6
  constraint perpendicular L5 L9
  constraint perpendicular L5 L8
  constraint perpendicular L8 L14
  constraint perpendicular L11 L14
  constraint perpendicular L2 L13
  constraint perpendicular L6 L10
  constraint perpendicular L2 L12
  constraint collinear L2 L9
  constraint tangent A18 L12
  constraint tangent L2 A18
  constraint tangent A5 L10
  constraint tangent A5 L12
  constraint equal A5 A18
  constraint tangent A8 L10
  constraint tangent L6 A8
  constraint equal A8 A18
  constraint tangent A6 L11
  constraint tangent A6 L13
  constraint tangent A19 L13
  constraint tangent L2 A19
  constraint equal A6 A19
  constraint tangent A4 L5
  constraint tangent A4 L8
  constraint equal A4 A6
  constraint tangent L5 A21
  constraint tangent L9 A21
  constraint equal A6 A21
  constraint tangent A1 L14
  constraint tangent A1 L11
  constraint equal A1 A6
  constraint tangent A3 L8
  constraint tangent A3 L14
  constraint equal A3 A6
  constraint tangent A2 L3
  constraint tangent A2 L9
  constraint equal A2 A6
  constraint tangent L0 A22
  constraint tangent L3 A22
  constraint equal A6 A22
  constraint tangent L0 A23
  constraint tangent L7 A23
  constraint equal A6 A23
  constraint horizontal L15
  constraint horizontal L4
  constraint horizontal L16
  constraint vertical L17
  constraint horizontal L18
  constraint vertical L19
  constraint horizontal L20
  constraint vertical L21
  constraint horizontal L22
  constraint vertical L23
  constraint horizontal L24
  constraint vertical L25
  constraint horizontal L26
  constraint vertical L27
  measures "d178" distance of origin P0
  measures "d179" diameter of A10
  measures "d180" diameter of A16
  measures "d181" diameter of A9
  measures "d182" diameter of A14
  measures "d183" diameter of A17
  measures "d184" diameter of A0
  measures "d185" diameter of A20
  measures "d186" diameter of A12
  measures "d190" radius of A18
  measures "d191" radius of A6
extrude "Extrude1" add sketch "Base Pieces" along normal blind 3 contours L0 L1 A4 L3 A11 L145 A112 L177 L178 A149 L448 L449 L450 L451 A233 A234 | A12 L4 A13 L5 L6 L7 L8 L9 L10 L11 A14 L12 L13 L28 L31 L35 L40 A35 L43 A39 A40 L45 L46 L47 L49 A103 L148 L157 L163 L164 L167 A119 L175 L176 A136 L181 L182 A146 L185 L187 L188 L189 L191 L193 L194 L195 A153 A155 L200 L202 A158 | A49 L54 L55 L56 L58 A54 L59 L60 L65 L67 A62 L78 A73 A74 L79 A75 L80 L81 L82 L83 L90 L91 L92 L94 L108 L110 L111 L115 L116 L120 A94 L126 L130 L132 L133 L135 L138 L144 L147 L152 L161 A127 A128 A134 | L204 L208 L210 L211 L212 L216 L217 L221 A175 L227 L231 L233 L234 L236 A179 A181 L239 L245 L249 A187 L254 L265 A206 A207 L284 A212 L285 A227 | L205 A186 L250 L261 L267 L268 L271 A198 L279 L282 A213 A214 L289 L290 A219 L293 L295 L296 L297 L299 L301 L302 L303 A224 A225 L309 L311 A228 | L246 A192 L283 L286 A221 L452 L453 L454 L455 A231 A232 makes body 1 at (190.092, 0, -77.3625) makes body 2 at (190.7467, 0, 143.3042) makes body 3 at (452.1308, 0, -183.3194) makes body 4 at (54.2968, 0, 38.3382) makes body 5 at (444.4899, 3, 43.0086) makes body 6 at (58.9385, 0, -189.0019)
extrude "Extrude2" add sketch "Base Pieces" along normal blind 3 separate body contours L0 L1 L2 A5 A9 L145 A133 L177 A139 L180 L448 L449 L450 L451 A233 A234 | L246 A211 L283 A215 L288 L452 L453 L454 L455 A231 A232 makes body 7 at (437.3959, 0, 191.5282) makes body 8 at (437.3959, 0, -28.4718)
extrude "Extrude3" add sketch "Top Shroud" along normal blind 3 separate body makes body 9
extrude "Extrude4" add sketch "Midplate LGP" along normal blind 3 separate body makes body 10
extrude "Extrude5" add sketch "PCB Backplate" along normal blind 3 separate body makes body 11
move_body "Move1" bodies 7 2 to x (1, 0, 0) y (0, 1, 0) z (0, 0, 1) at (-100, 0, -220)
move_body "Move2" bodies 1 8 to x (1, 0, 0) y (0, 1, 0) z (0, 0, 1) at (-100, 3, 0)
move_body "Move3" bodies 11 to x (1, 0, 0) y (0, 1, 0) z (0, 0, 1) at (0, 6, 0)
other "Modify15"
move_body "Move4" bodies 10 to x (1, 0, 0) y (0, 1, 0) z (0, 0, 1) at (0, 10.5, 0)
move_body "Move5" bodies 9 to x (1, 0, 0) y (0, 1, 0) z (0, 0, 1) at (0, 13.5, 0)
sketch "TouchFilm_Size_DimensionsFixed" plane through (0, 0, 0) normal (0, 1, 0) x (1, 0, 0)
  arc A0 (492.3492, 109.375) -> (497.9874, 105.4271) centre (492.3492, 103.375) cw
  line L0 (513.6381, 58.3229) -> (497.9874, 15.3229)
  line L1 (15.697, 109.375) -> (484.303, 109.375)
  line L2 (484.3058, 11.375) -> (15.6942, 11.375)
  arc A1 (-13.6381, 58.3229) -> (-13.6381, 62.4271) centre (-7.9999, 60.375) cw
  line L3 (484.303, 109.375) -> (492.3492, 109.375)
  line L4 (7.6508, 109.375) -> (15.697, 109.375)
  line L5 (2.0126, 15.3229) -> (-13.6381, 58.3229)
  line L6 (-13.6381, 62.4271) -> (2.0126, 105.4271)
  line L7 (497.9874, 105.4271) -> (513.6381, 62.4271)
  arc A2 (2.0126, 105.4271) -> (7.6508, 109.375) centre (7.6508, 103.375) cw
  line L8 (492.3492, 11.375) -> (484.3058, 11.375)
  arc A3 (513.6381, 62.4271) -> (513.6381, 58.3229) centre (507.9999, 60.375) cw
  arc A4 (7.6508, 11.375) -> (2.0126, 15.3229) centre (7.6508, 17.375) cw
  line L9 (15.6942, 11.375) -> (7.6508, 11.375)
  arc A5 (497.9874, 15.3229) -> (492.3492, 11.375) centre (492.3492, 17.375) cw
hidden bodies 3 4 5 6
equation "d157 = ( 5.5 / 2 ) * 1 mm"
equation "d158 = ( 5.5 / 2 ) * 1 mm"
equation "d159 = ( 5.5 / 2 ) * 1 mm"
equation "d160 = ( 5.5 / 2 ) * 1 mm"
equation "d161 = ( 5.5 / 2 ) * 1 mm"
equation "d162 = ( 5.5 / 2 ) * 1 mm"
equation "d163 = ( 5.5 / 2 ) * 1 mm"
equation "d164 = ( 5.5 / 2 ) * 1 mm"
equation "d165 = ( 5.5 / 2 ) * 1 mm"
equation "d166 = ( 5.5 / 2 ) * 1 mm"
equation "d167 = ( 5.5 / 2 ) * 1 mm"
named bodies: "Base 3", "Base 1", "Base 2", "Base 4", "Top Shroud", "Midplane LGP", "PCB Backplane"
